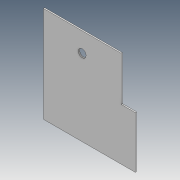
# Autodesk Inventor part: tampa
Saved by Autodesk Inventor 2021 (Build 250183000, 183)
## iProperties
Created: 2020-10-16
Part Number: tampa
Material: Genérico
Document SubType Name: Modeling
Designer: evert
Density: 1 g/cm^3
Appearance: Padrão
Author: evert
Autodesk Inventor part; units mm, degrees
ref_plane "YZ Plane" through (0, 0, 0) normal (1, 0, 0) x (0, 1, 0)
ref_plane "XZ Plane" through (0, 0, 0) normal (0, 1, 0) x (-1, 0, 0)
ref_plane "XY Plane" through (0, 0, 0) normal (0, 0, 1) x (1, 0, 0)
sketch "Esboço1" plane through (0, 0, 0) normal (0, 0, 1) x (1, 0, 0)
  line L0 (0, 0) -> (30, 0)
  line L1 (30, 0) -> (30, -36.4)
  line L2 (30, -36.4) -> (0, -36.4)
  line L3 (0, -36.4) -> (0, 0)
  dimension "d0" = 30
  dimension "d1" = 36.4
  constraints: 8 end point, 2 parallel, 1 horizontal, 1 perpendicular
  measures "d0" distance of L1.end L2.end
  measures "d1" distance of L0.end L1.end
extrude "Extrusão1" add sketch "Esboço1" along normal blind 0.5
sketch "Esboço2" plane through (0, 0, 0.5) normal (0, 0, 1) x (1, 0, 0)
  line L0 (30, 0) -> (0, 0) projected
  line L1 (0, 0) -> (15, 0)
  line L2 (15, 0) -> (15, -7.5)
  circle A0 centre (15, -7.5) radius 1.5
  dimension "d4" = 7.5
  dimension "d5" = 3
  constraints: 4 end point, 1 centre point, 1 coincident, 1 midpoint, 1 perpendicular
  measures "d4" distance of L1.end L2.end
  measures "d5" diameter of A0
extrude "Extrusão2" cut sketch "Esboço2" against normal blind 0.5
sketch "Esboço4" plane through (0, 0, 0.5) normal (0, 0, 1) x (1, 0, 0)
  line L0 (0, -36.4) -> (30, -36.4) projected
  line L1 (0, -36.4) -> (30, -36.4)
  line L2 (30, -36.4) -> (30, -37.1)
  line L3 (30, -37.1) -> (0, -37.1)
  line L4 (0, -37.1) -> (0, -36.4)
  point P0 (0, 0)
  dimension "d10" = 0.7
  constraints: 8 end point, 2 parallel, 1 horizontal, 1 perpendicular
  measures "d10" distance of L1.end L2.end
extrude "Extrusão3" add sketch "Esboço4" against normal blind 0.5
sketch "Esboço5" plane through (0, 0, 0.5) normal (0, 0, 1) x (1, 0, 0)
  line L0 (0, 0) -> (0, -37.1) projected
  line L1 (0, -37.1) -> (4, -37.1)
  line L2 (30, -37.1) -> (0, -37.1) projected
  line L3 (30, -37.1) -> (30, 0) projected
  line L4 (30, -37.1) -> (26, -37.1)
  line L5 (30, -37.1) -> (35.5, -37.1)
  line L6 (35.5, -37.1) -> (35.5, -17.1)
  line L7 (35.5, -17.1) -> (30, -17.1)
  dimension "d13" = 4
  dimension "d14" = 4
  dimension "d15" = 5.5
  dimension "d16" = 20
  constraints: 10 end point, 3 point on line, 2 perpendicular, 1 horizontal
  measures "d13" distance of L0.end L1.end
  measures "d14" distance of L2.start L4.end
  measures "d15" distance of L2.start L5.end
  measures "d16" distance of L5.end L6.end
extrude "Extrusão4" add sketch "Esboço5" against normal blind 0.5
